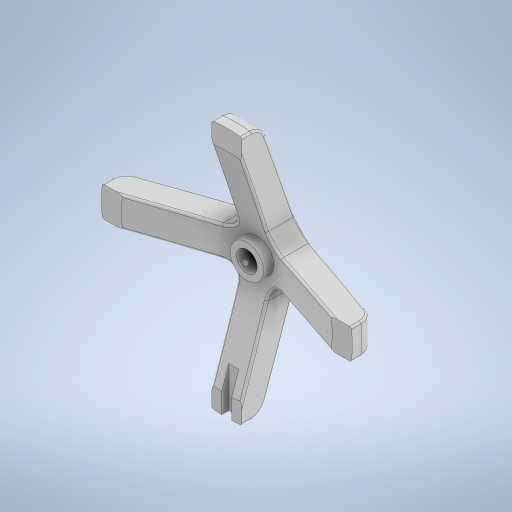
# Autodesk Inventor part: Pie
Saved by Autodesk Inventor 2024 (Build 280153000, 153)
## iProperties
Created: 2023-11-25
Part Number: Pie
Material: Genérico
Document SubType Name: Modeling
Designer: sergi
Density: 1 g/cm^3
Appearance: Valor por defecto
Author: sergi
Autodesk Inventor part; units mm, degrees
ref_plane "YZ Plane" through (0, 0, 0) normal (1, 0, 0) x (0, 1, 0)
ref_plane "XZ Plane" through (0, 0, 0) normal (0, 1, 0) x (-1, 0, 0)
ref_plane "XY Plane" through (0, 0, 0) normal (0, 0, 1) x (1, 0, 0)
sketch "Boceto1" plane through (0, 0, 0) normal (0, 0, 1) x (1, 0, 0)
  circle A0 centre (0, 0) radius 125
  dimension "d0" = 250
  constraints: 1 centre point, 1 coincident
  measures "d0" diameter of A0
extrude "Extrusión1" add sketch "Boceto1" along normal blind 20
sketch "Boceto3" plane through (0, 0, 0) normal (0, 0, -1) x (-1, 0, 0)
  circle A0 centre (0, 0) radius 125 projected
  circle A1 centre (0, 0) radius 10.05 projected
  circle A2 centre (0, 0) radius 7.1 projected
  circle A3 centre (0, 0) radius 9.1 projected
  circle A4 centre (0, 0) radius 9.6 projected
  circle A5 centre (0, 0) radius 10.3
  dimension "d6" = 0.25
  constraints: 1 centre point
  measures "d6" radial gap between concentric circles of A1 A5
extrude "Extrusión3" add sketch "Boceto3" along normal blind 40 contours A0
chamfer "Chaflán1" distance 112 distance2 40 1 edges at (125, 0, -40) measured on face at (124.5, 0, -40)
sketch "Boceto4" plane through (0, 0, 20) normal (0, 0, 1) x (1, 0, 0)
  circle A0 centre (0, 0) radius 125 projected
  constraints: 1 coincident
hole "Agujero1" at (0, 0, 20) direction (0, 0, -1) diameter 10 end through all
sketch "Boceto5" plane through (0, 0, 20) normal (0, 0, 1) x (1, 0, 0)
  circle A0 centre (0, 0) radius 5 projected
  line L0 (-5, 0) -> (5, 0)
  line L1 (5, 0) -> (5, -133.872)
  line L2 (5, -133.872) -> (-5, -133.872)
  line L3 (-5, -133.872) -> (-5, 0)
  dimension "d19" = 10
  constraints: 8 end point, 2 parallel, 1 horizontal, 1 perpendicular, 2 other
  measures "d19" distance of L1.end L2.end
extrude "Extrusión4" cut sketch "Boceto5" against normal blind 7 contours L1 L2 L3 A0
sketch "Boceto6" plane through (0, 0, 20) normal (0, 0, 1) x (1, 0, 0)
  line L0 (0, 0) -> (142.9455, 0)
  line L1 (0, -15) -> (142.9455, -15)
  line L2 (0, 15) -> (142.9455, 15)
  line L3 (0, 0) -> (0, -153.4537)
  line L4 (15, 0) -> (15, -153.4537)
  line L5 (-15, 0) -> (-15, -153.4537)
  line L6 (15, 0) -> (15, 189.8366)
  line L7 (-15, 0) -> (-15, 175.0031)
  line L8 (0, 15) -> (-140.708, 15)
  line L9 (0, -15) -> (-140.708, -15)
  line L10 (-5, -124.9) -> (-5, 0) projected
  arc A0 (5, 0) -> (-5, 0) centre (0, 0) ccw projected
  line L11 (5, 0) -> (5, -124.9) projected
  arc A1 (5, -124.9) -> (-5, -124.9) centre (0, 0) ccw projected
  point P0 (-15, 124.0967)
  point P1 (-124.0967, 15)
  point P2 (-15, 15)
  point P3 (-124.0967, -15)
  point P4 (-15, -124.0967)
  point P5 (-15, -15)
  point P6 (15, -124.0967)
  point P7 (124.0967, -15)
  point P8 (15, -15)
  point P9 (124.0967, 15)
  point P10 (15, 124.0967)
  point P11 (15, 15)
  dimension "d22" = 15
  dimension "d23" = 30
  dimension "d24" = 15
  dimension "d25" = 30
  constraints: 20 end point, 4 parallel, 3 horizontal, 3 vertical
  measures "d22" distance between parallel lines of L0 L1
  measures "d23" distance between parallel lines of L1 L2
  measures "d24" distance between parallel lines of L3 L4
  measures "d25" distance between parallel lines of L4 L5
extrude "Extrusión5" cut sketch "Boceto6" against normal through all contours L1 A1 L4 | L6 A1 L2 | L5 A1 L9 | L8 A1 L7
sketch "Boceto7" plane through (0, 0, 20) normal (0, 0, 1) x (1, 0, 0)
  arc A0 (5, 0) -> (-5, 0) centre (0, 0) ccw projected
  circle A1 centre (0, 0) radius 125
  circle A2 centre (0, 0) radius 105
  dimension "d28" = 20
  constraints: 2 centre point, 1 coincident
  measures "d28" radial gap between concentric circles of A1 A2
sketch "Boceto8" plane through (15, 15, 20) normal (1, 0, 0) x (0, 0, -1)
  line L0 (0, 109.0967) -> (20, 109.0967) projected
  line L1 (0, 0) -> (0, 109.0967) projected
  line L2 (0, 0) -> (57.0667, 0) projected
  line L3 (20, 109.0967) -> (20, 0)
  line L4 (20, 109.0967) -> (57.0667, 0)
  point P0 (20, -15)
  dimension "d29" = 18.766
  constraints: 4 end point, 1 perpendicular, 1 point on line, 1 other
  measures "d29" angle of L3 L4
extrude "Extrusión6" cut sketch "Boceto7" against normal blind 30 draft -71.23 contours A2
sketch "Boceto9" plane through (-15, -124.0967, 0) normal (-1, 0, 0) x (0, 0, 1)
  line L0 (-8.4744, 109.0967) -> (-37.0667, 109.0967) projected
  line L1 (20, 0) -> (0, 0) projected
  line L2 (20, 20.1737) -> (20, 0) projected
  line L3 (0, 0) -> (-37.0667, 109.0967)
  line L4 (24.0751, 8.1797) -> (-12.9917, 117.2765)
  point P0 (0, 124.0967)
  dimension "d32" = 25.4267
  constraints: 4 end point, 1 parallel, 2 other
  measures "d32" distance between parallel lines of L4 L3
sketch "Boceto10" plane through (0, 0, -10) normal (0, 0, 1) x (1, 0, 0)
  circle A0 centre (0, 0) radius 10.3 projected
  circle A1 centre (0, 0) radius 16.7241 projected
extrude "Extrusión7" add sketch "Boceto10" along normal blind 10
sketch "Boceto11" plane through (0, 0, 0) normal (0, 0, 1) x (1, 0, 0)
  line L0 (0, 0) -> (-39.9996, 39.9996)
  line L1 (0, 0) -> (56.5679, 0) construction
  circle A0 centre (0, 0) radius 16.7241 projected
  circle A1 centre (0, 0) radius 10.3 projected
  dimension "d35" = 135
  constraints: 4 end point, 1 equal length, 1 horizontal
  measures "d35" angle of L1 L0
ref_plane "Plano de trabajo1" through (0, 0, 0) normal (0.7071068, 0.7071068, 0) x (-0.7071068, 0.7071068, 0)
sketch "Boceto12" plane through (0, 0, 0) normal (0.7071068, 0.7071068, 0) x (-0.7071068, 0.7071068, 0)
  line L0 (16.7241, 0) -> (-16.7241, 0) projected
  line L1 (16.7241, -10) -> (-16.7241, -10) projected
  line L2 (0, -10) -> (0, 0)
  circle A0 centre (0, -5) radius 3.2
  dimension "d37" = 6.4
  constraints: 2 end point, 2 midpoint, 1 centre point, 1 vertical
  measures "d37" diameter of A0
extrude "Extrusión8" cut sketch "Boceto12" against normal through all
fillet "Empalme1" radius 15 5 edges at (0, -125, -0.0001) (-124.774, 7.5136, -0.0001) (-124.774, -7.5136, -0.0001) (0, 125, 0) (125, 0, -0.0001)
fillet "Empalme2" radius 15 4 edges at (-15, -15, -22.7706) (-15, 15, -22.7706) (15, 15, -22.7706) (15, -15, -22.7706)
fillet "Empalme3" radius 2 40 edges at (-19.3933, 19.3935, -34.8478) (-15, 59.3954, -22.7643) (-15, 121.3317, 1.9217) (-15, 124.0967, 15.2853) (-121.324, 15, 1.9109) (-124.0967, 15, 15.2853) (-59.3954, 15, -22.7643) (19.3933, 19.3935, -34.8478) (59.3954, 15, -22.7643) (121.3317, 15, 1.9217) (124.0967, 15, 15.2853) (15, 121.3317, 1.9217) (15, 124.0967, 15.2853) (15, 59.3954, -22.7643) (19.3933, -19.3935, -34.8478) (15, -59.3954, -22.7643) (15, -121.3317, 1.9217) (15, -124.0967, 15.2853) (121.3317, -15, 1.9217) (124.0967, -15, 15.2853) (59.3954, -15, -22.7643) (-19.3933, -19.3935, -34.8478) (-59.3954, -15, -22.7643) (-121.324, -15, 1.9109) (-124.0967, -15, 15.2853) (-15, -121.3317, 1.9217) (-15, -124.0967, 15.2853) (-15, -59.3954, -22.7643) (19.3933, 19.3935, -6.3629) (15, 56.6326, 4.2263) (56.6326, 15, 4.2263) (-19.3933, 19.3935, -6.3629) (-56.6326, 15, 4.2263) (-15, 56.6326, 4.2263) (19.3933, -19.3935, -6.3629) (56.6326, -15, 4.2263) (15, -56.6326, 4.2263) (-19.3933, -19.3935, -6.3629) (-56.6326, -15, 4.2263) (-15, -56.6326, 4.2263)
